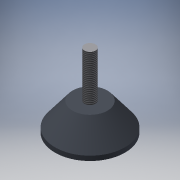
# Autodesk Inventor part: 21-013
Saved by Autodesk Inventor 2018 (Build 220105000, 105)
## iProperties
Shininess: 64.0
Length Units: 11269
Angle Units: 11279
Time Units: 11290
Mass Units: 11286
Length Display Precision: 3
Angle Display Precision: 2
Compacted: True
Created: 2003-01-06
Part Number: 21-013
Vendor: PARKER IPS
Document SubType Name: Modeling
Designer: Autodesk, Inc.
Description: KNUCKLE FOOT 80, M12x80
Catalog Web Link: http://www.parker.com/ead/cm1.asp?cmid=809
Mass: 39.8452 g
Surface Area: 167.331 cm^2
Volume: 39.8452 cm^3
Density: 1 g/cm^3
Material: Generic
Appearance: Default
Density: 0.0
Volumn: 0.0
Area: 0.0
PropertySet Name: Model Information
Control State: 0
Master: False
Checked Out: False
CAGE: 08JJ3
NEXT HIGHER ASSY 01: ---
Author: Autodesk, Inc.
Autodesk Inventor part; units mm, degrees
ref_plane "YZ Plane" through (0, 0, 0) normal (1, 0, 0) x (0, 1, 0)
ref_plane "XZ Plane" through (0, 0, 0) normal (0, 1, 0) x (-1, 0, 0)
ref_plane "XY Plane" through (0, 0, 0) normal (0, 0, 1) x (1, 0, 0)
sketch "Sketch1" plane through (0, 0, 0) normal (0, 0, 1) x (1, 0, 0)
  line L0 (0, 0) -> (0, 30)
  line L1 (0, 30) -> (19, 30)
  line L2 (19, 30) -> (38, 5)
  line L3 (38, 5) -> (38, 0)
  line L4 (38, 0) -> (0, 0)
  dimension "C" = 76
  dimension "d1" = 30
  dimension "d2" = 5
  dimension "d3" = 38
  constraints: 10 end point, 2 parallel, 1 perpendicular, 1 vertical, 1 other
  measures "C" diameter of L3 L0
  measures "d1" distance of L0.start L0.end
  measures "d2" distance of L2.end L3.end
  measures "d3" diameter of L1.end L0
revolve "Revolution1" add sketch "Sketch1" angle 360 about axis through (0, 0, 0) along (0, 1, 0)
shell "Shell1" thickness 5 removed faces 1 at (9.1519, 0, -15.3991)
sketch "Sketch2" plane through (0, 30, 0) normal (0, 1, 0) x (1, 0, 0)
  circle A0 centre (0, 0) radius 19 projected
  circle A1 centre (0, 0) radius 6
  dimension "d6" = 12
  constraints: 1 centre point, 1 coincident
  measures "d6" diameter of A1
extrude "Extrusion1" add sketch "Sketch2" along normal blind 50 contours A1
thread "Thread1" size "M12x1.75" class "6g" standard "ANSI Metric M Profile" full length
equation "\"d3\" = 0.5 * C"
equation "\"d7\" = Dmax - d1"
equation "\"Dmin\" = 41"
equation "\"Dmax\" = 80"
body "Solid1"
